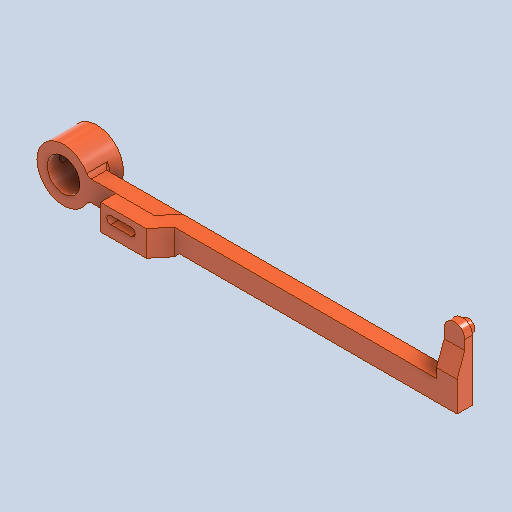
# Autodesk Inventor part: head_lock_2
Saved by Autodesk Inventor 2024 (Build 280153000, 153)
## iProperties
Created: 2021-06-14
Part Number: head_lock_2
Material: Generic
Document SubType Name: Modeling
Designer: dsdan
Density: 1 g/cm^3
Appearance: Smooth - Light Orange
Author: dsdan
Autodesk Inventor part; units mm, degrees
ref_plane "YZ Plane" through (0, 0, 0) normal (1, 0, 0) x (0, 1, 0)
ref_plane "XZ Plane" through (0, 0, 0) normal (0, 1, 0) x (-1, 0, 0)
ref_plane "XY Plane" through (0, 0, 0) normal (0, 0, 1) x (1, 0, 0)
sketch "Sketch1" plane through (0, 0, 0) normal (0, 0, 1) x (1, 0, 0)
  circle A0 centre (7.9364, -24.4124) radius 2.575 construction
  circle A1 centre (7.9364, -24.4124) radius 2.55
  dimension "d70" = 5.1
  constraints: 1 centre point, 1 coincident
  measures "d70" diameter of A1
extrude "Extrusion1" add sketch "Sketch1" against normal blind 2.4
sketch "Sketch2" plane through (0, 0, 0) normal (0, 0, 1) x (1, 0, 0)
  arc A0 (11.9364, -24.4124) -> (3.9364, -24.4124) centre (7.9364, -24.4124) ccw
  line L0 (11.9364, -24.4124) -> (3.9364, -24.4124) construction
  line L1 (3.9364, -24.4124) -> (3.9364, -40.0897)
  line L2 (11.9364, -48.0897) -> (11.9364, -24.4124)
  line L3 (-141.4747, -48.1269) -> (-141.4747, -40.1269) construction
  line L4 (-131.9289, -40.0897) -> (3.9364, -40.0897)
  arc A1 (-131.9289, -40.0897) -> (-131.9289, -48.0897) centre (-141.4747, -44.0897) ccw
  line L5 (11.9364, -48.0897) -> (-131.9289, -48.0897)
  circle A2 centre (-141.4747, -44.0897) radius 6.35
  line L6 (-118.5278, -40.0897) -> (-118.5278, -48.0897) construction
  circle A3 centre (-141.4747, -44.0897) radius 5.8293 projected
  circle A4 centre (7.9364, -24.4124) radius 2.55 projected
  point P0 (-118.5278, -44.0897)
  point P1 (12.7405, -19.0124)
  dimension "d3" = 8
  dimension "d36" = 12.7
  dimension "d37" = 4
  dimension "d38" = 8
  constraints: 14 end point, 4 point on circle, 3 centre point, 3 coincident, 3 perpendicular, 3 point on line, 2 horizontal, 2 parallel, 2 tangent, 1 concentric, 1 horizontal alignment, 1 midpoint, 1 other
  measures "d3" diameter of A0
  measures "d36" diameter of A2
  measures "d37" radial gap between concentric circles of A1 A2
  measures "d38" distance between parallel lines of L5 L4
extrude "Extrusion2" add sketch "Sketch2" along normal blind 6 contours L2 L5 A1 L4 L1 A0 | A4
sketch "Sketch3" plane through (3.9364, -40.0897, 0) normal (-1, 0, 0) x (0, 0, 1)
  line L0 (0, 19.6772) -> (6, 19.6772) projected
  line L1 (3, 19.6772) -> (3, 11.9197)
  line L2 (3, 11.9197) -> (6, 3.6772)
  line L3 (6, 15.6772) -> (6, 19.6772) projected
  line L4 (6, 15.6772) -> (6, 0) projected
  point P0 (0, 40.0897)
  point P1 (5, 8)
  dimension "d8" = 160
  dimension "d10" = 16
  constraints: 4 end point, 1 midpoint, 1 perpendicular, 2 other
  measures "d8" angle of L1 L2
  measures "d10" distance of L0.end L2.end
extrude "Extrusion3" cut sketch "Sketch3" against normal through all
ref_plane "Work Plane3" through (-155.9002, -65.296, -7) normal (0, 0, 1) x (1, 0, 0)
sketch "Sketch8" plane through (-124.0334, -23.6772, 0) normal (0, 0, 1) x (1, 0, 0)
  arc A0 (-7.8955, -16.4124) -> (-7.8955, -24.4124) centre (-17.4413, -20.4124) ccw projected
  circle A1 centre (-17.4413, -20.4124) radius 6.35 projected
  circle A2 centre (-17.4413, -20.4124) radius 10.35
  point P0 (124.0334, 23.6772)
  point P1 (-7.8955, -24.4124)
  point P2 (-7.8955, -16.4124)
  constraints: 1 centre point, 1 coincident, 1 concentric
extrude "Extrusion8" add sketch "Sketch8" against normal up to surface (7 mm away)
fillet "Fillet1" radius 2 3 edges at (-131.1247, -44.0897, 0) (-131.9289, -48.0897, 3) (-131.9289, -40.0897, 3)
ref_plane "Work Plane2" through (-151.8247, -44.0897, 0) normal (-1, 0, 0) x (0, 0, 1)
sketch "Sketch9" plane through (-151.8247, -44.0897, 0) normal (-1, 0, 0) x (0, 0, 1)
  circle A0 centre (-0.5, 0) radius 1.8
  line L0 (6, -10.35) -> (6, 10.35) projected
  point P0 (0, 44.0897)
  point P1 (6, 5.0283)
  point P2 (6, -5.0283)
  point P3 (6, 0)
  dimension "d31" = 3.6
  dimension "d41" = 6.5
  constraints: 1 centre point, 1 horizontal alignment, 1 midpoint
  measures "d31" diameter of A0
  measures "d41" distance from line of A0.centre L0
extrude "Extrusion9" cut sketch "Sketch9" against normal up to next
sketch "Sketch10" plane through (11.9364, -48.0897, 0) normal (0, -1, 0) x (1, 0, 0)
  line L0 (-8, 6) -> (-142.6166, 6) projected
  line L1 (-118, 6) -> (-113, 0)
  line L2 (-8, 0) -> (-141.7268, 0) projected
  point P0 (-11.9364, 0)
  point P1 (-142.6169, 0)
  point P2 (-143.7603, 0)
  constraints: 2 end point, 2 point on line
surface extrude "ExtrusionSrf1" sketch "Sketch10" against normal through all shown no curves L1
split body "Split1" result two bodies by surface "ExtrusionSrf1" first body at (-134.0139, -50.5208, -1)
sketch "Sketch11" plane through (11.9364, -48.0897, 0) normal (0, -1, 0) x (1, 0, 0)
  line L0 (-8, 6) -> (-118, 6) projected
  line L1 (-110.1898, 6) -> (-115.1898, 12)
  line L2 (-110.1898, 6) -> (-102.3795, 6) construction
  line L3 (-115.1898, 12) -> (-133, 12)
  line L4 (-133, 12) -> (-133, 6)
  line L5 (-142.6166, 6) -> (-118, 6) projected
  line L6 (-133, 6) -> (-118, 6)
  line L7 (-118, 6) -> (-113, 0) projected
  line L8 (-118, 6) -> (-110.1898, 6)
  line L9 (-113, 0) -> (-141.7268, 0) projected
  line L10 (-113, 0) -> (0, 0) projected
  point P0 (-11.9364, 0)
  point P1 (-142.6169, 0)
  point P2 (-143.7603, 0)
  dimension "d47" = 6
  dimension "d48" = 6
  dimension "d49" = 15
  dimension "d64" = 6
  constraints: 12 end point, 2 horizontal, 1 collinear, 1 equal length, 1 parallel, 1 perpendicular, 1 point on line
  measures "d47" vertical distance of L1.start L1.end
  measures "d48" distance between parallel lines of L7 L1
  measures "d49" distance from line of L0.end L4
  measures "d64" distance between parallel lines of L10 L0
extrude "Extrusion10" add sketch "Sketch11" against normal up to surface (8 mm away) bodies 3
sketch "Sketch12" plane through (-121.0636, -48.0897, 12) normal (0, 0, 1) x (1, 0, 0)
  line L0 (4, 4) -> (12, 4) construction
  line L1 (4, 2.45) -> (12, 2.45)
  line L2 (12, 5.55) -> (4, 5.55)
  arc A0 (4, 5.55) -> (4, 2.45) centre (4, 4) ccw
  arc A1 (12, 2.45) -> (12, 5.55) centre (12, 4) ccw
  line L3 (0, 0) -> (0, 8) projected
  line L4 (17.8102, 0) -> (17.8102, 8) projected
  point P0 (121.0636, 48.0897)
  point P1 (8, 4)
  point P2 (0, 4)
  dimension "d52" = 8
  dimension "d53" = 3.1
  dimension "d54" = 4
  constraints: 8 end point, 4 point on circle, 4 tangent, 2 centre point, 2 midpoint, 1 horizontal, 1 parallel, 1 point on line
  measures "d52" distance of L0.start L0.end
  measures "d53" diameter of A1
  measures "d54" distance from line of L3 L0.start
extrude "Extrusion11" cut sketch "Sketch12" against normal through all bodies 3
sketch "Sketch13" plane through (0, 0, 6) normal (0, 0, 1) x (1, 0, 0)
  arc A0 (-109.0636, -45.6397) -> (-109.0636, -42.5397) centre (-109.0636, -44.0897) ccw projected
  circle A1 centre (-109.0636, -44.0897) radius 2.4
  point P0 (0, 0)
  dimension "d58" = 4.8
  constraints: 1 centre point, 1 coincident
  measures "d58" diameter of A1
extrude "Extrusion12" cut sketch "Sketch13" against normal through all bodies 2
chamfer "Chamfer1" distance 0.5 angle 45 1 edges at (-111.4636, -44.0897, 0)
sketch "Sketch14" plane through (11.9364, -48.0897, 0) normal (0, -1, 0) x (1, 0, 0)
  line L0 (-115.1898, 12) -> (-133, 12) projected
  line L1 (-133, 12) -> (-115.1898, 12)
  line L2 (-133, 0) -> (-133, 12)
  line L3 (-110.1898, 6) -> (-115.1898, 12) projected
  line L4 (-115.1898, 12) -> (-110.1898, 6)
  line L5 (-110.1898, 0) -> (-110.1898, 6)
  line L6 (-141.7268, 0) -> (-113, 0) projected
  line L7 (-133, 0) -> (-110.1898, 0)
  point P0 (-11.9364, 0)
  point P1 (-142.6169, 0)
  point P2 (-143.7603, 0)
  constraints: 10 end point, 3 point on line, 2 collinear, 1 horizontal, 1 perpendicular, 1 vertical
extrude "Extrusion13" add sketch "Sketch14" along normal blind 2 bodies 3
chamfer "Chamfer2" distance 2 angle 45 1 edges at (-98.2533, -48.0897, 3)
equation "\"d47\" = d64"
equation "\"d48\" = d47"
body "Srf1"
body "Solid2"
body "Solid3"
